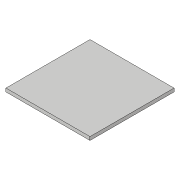
# Autodesk Inventor part: Electronics Container Part 1
Saved by Autodesk Inventor 2018.3 (Build 223284000, 284)
## iProperties
Created: 2019-03-04
Part Number: Electronics Container Part 1
Material: Generic
Document SubType Name: Modeling
Designer: aye06091
Mass: 20.0037 g
Surface Area: 136.088 cm^2
Volume: 20.0037 cm^3
Density: 1 g/cm^3
Appearance: Default
Author: aye06091
Autodesk Inventor part; units mm, degrees
ref_plane "YZ Plane" through (0, 0, 0) normal (1, 0, 0) x (0, 1, 0)
ref_plane "XZ Plane" through (0, 0, 0) normal (0, 1, 0) x (-1, 0, 0)
ref_plane "XY Plane" through (0, 0, 0) normal (0, 0, 1) x (1, 0, 0)
sketch "Sketch1" plane through (0, 0, 0) normal (0, 1, 0) x (-1, 0, 0)
  line L0 (0, 0) -> (-79.375, 0)
  line L1 (-79.375, 0) -> (-79.375, 79.375)
  line L2 (-79.375, 79.375) -> (0, 79.375)
  line L3 (0, 79.375) -> (0, 0)
  dimension "d0" = 79.375
  dimension "d1" = 79.375
  constraints: 8 end point, 2 parallel, 1 horizontal, 1 perpendicular
  measures "d0" distance of L0.start L0.end
  measures "d1" distance of L2.end L0.start
extrude "Extrusion1" add sketch "Sketch1" against normal blind 3.175
body "Solid1"
